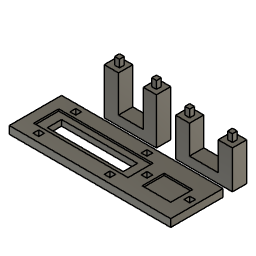
finalFrame_v1 (Autodesk Fusion 360 design; units mm, degrees)
Autodesk Fusion 360 part; units mm, degrees
sketch "草图1" plane through (0, 0, 0) normal (0, 0, 1) x (1, 0, 0)
  line L0 (0, 0) -> (-99.2, 0)
  line L1 (-99.2, 0) -> (-99.2, 26.2)
  line L2 (-99.2, 26.2) -> (0, 26.2)
  line L3 (0, 26.2) -> (0, 0)
  line L4 (15, 0) -> (45, 0)
  line L5 (45, 0) -> (45, 23)
  line L6 (45, 23) -> (15, 23)
  line L7 (15, 23) -> (15, 0)
  line L8 (5, 15) -> (10, 15)
  line L9 (10, 15) -> (10, 10)
  line L10 (10, 10) -> (5, 10)
  line L11 (5, 10) -> (5, 15)
  line L12 (50, 15) -> (55, 15)
  line L13 (55, 15) -> (55, 10)
  line L14 (55, 10) -> (50, 10)
  line L15 (50, 10) -> (50, 15)
  line L16 (-90, 35) -> (-85, 35)
  line L17 (-85, 35) -> (-85, 30)
  line L18 (-85, 30) -> (-90, 30)
  line L19 (-90, 30) -> (-90, 35)
  line L20 (-90, -4) -> (-85, -4)
  line L21 (-85, -4) -> (-85, -9)
  line L22 (-85, -9) -> (-90, -9)
  line L23 (-90, -9) -> (-90, -4)
  line L24 (-15, 35) -> (-10, 35)
  line L25 (-10, 35) -> (-10, 30)
  line L26 (-10, 30) -> (-15, 30)
  line L27 (-15, 30) -> (-15, 35)
  line L28 (-15, -9) -> (-10, -9)
  line L29 (-10, -9) -> (-10, -4)
  line L30 (-10, -4) -> (-15, -4)
  line L31 (-15, -4) -> (-15, -9)
  line L32 (-110, 40) -> (60, 40)
  line L33 (60, 40) -> (60, -15)
  line L34 (60, -15) -> (-110, -15)
  line L35 (-110, -15) -> (-110, 40)
  line L36 (-90, 20) -> (-10, 20)
  line L37 (-10, 20) -> (-10, 5)
  line L38 (-10, 5) -> (-90, 5)
  line L39 (-90, 5) -> (-90, 20)
  dimension "d1" = 26.2
  dimension "d2" = 99.2
  dimension "d3" = 23
  dimension "d4" = 30
  dimension "d5" = 5
  dimension "d6" = 5
  dimension "d7" = 55
  dimension "d8" = 170
  constraint horizontal L0
  constraint vertical L1
  constraint horizontal L2
  constraint vertical L3
  constraint coincident L0.start L3.end
  constraint horizontal L4
  constraint vertical L5
  constraint horizontal L6
  constraint vertical L7
  constraint horizontal L8
  constraint vertical L9
  constraint horizontal L10
  constraint vertical L11
  constraint horizontal L12
  constraint vertical L13
  constraint horizontal L14
  constraint vertical L15
  constraint horizontal L16
  constraint vertical L17
  constraint horizontal L18
  constraint vertical L19
  constraint horizontal L20
  constraint vertical L21
  constraint horizontal L22
  constraint vertical L23
  constraint horizontal L24
  constraint vertical L25
  constraint horizontal L26
  constraint vertical L27
  constraint horizontal L28
  constraint vertical L29
  constraint horizontal L30
  constraint vertical L31
  constraint horizontal L32
  constraint vertical L33
  constraint horizontal L34
  constraint vertical L35
  constraint horizontal L36
  constraint vertical L37
  constraint horizontal L38
  constraint vertical L39
  measures "d1" distance of L0.end L1.end
  measures "d2" distance of L1.end L2.end
  measures "d3" distance of L4.end L5.end
  measures "d4" distance of L5.end L6.end
  measures "d5" distance of L12.start L14.end
  measures "d6" distance of L12.start L12.end
  measures "d7" distance of L32.start L34.end
  measures "d8" distance of L32.start L32.end
sketch "草图2" plane through (0, 0, 0) normal (0, 0, 1) x (1, 0, 0)
  line L0 (-90, -9) -> (-85, -9)
  line L1 (-85, -9) -> (-85, -4)
  line L2 (-85, -4) -> (-90, -4)
  line L3 (-90, -4) -> (-90, -9)
  line L4 (-15, -9) -> (-10, -9)
  line L5 (-10, -9) -> (-10, -4)
  line L6 (-10, -4) -> (-15, -4)
  line L7 (-15, -4) -> (-15, -9)
  line L8 (-15, 30) -> (-10, 30)
  line L9 (-10, 30) -> (-10, 35)
  line L10 (-10, 35) -> (-15, 35)
  line L11 (-15, 35) -> (-15, 30)
  line L12 (-90, 30) -> (-85, 30)
  line L13 (-85, 30) -> (-85, 35)
  line L14 (-85, 35) -> (-90, 35)
  line L15 (-90, 35) -> (-90, 30)
  line L16 (-95, 26.2) -> (-80, 26.2)
  line L17 (-80, 26.2) -> (-80, 40)
  line L18 (-80, 40) -> (-95, 40)
  line L19 (-95, 40) -> (-95, 26.2)
  line L20 (-95, -15) -> (-80, -15)
  line L21 (-80, -15) -> (-80, 0)
  line L22 (-80, 0) -> (-95, 0)
  line L23 (-95, 0) -> (-95, -15)
  line L24 (-95, -15) -> (-80, -15)
  line L25 (-80, -15) -> (-80, 40)
  line L26 (-80, 40) -> (-95, 40)
  line L27 (-95, 40) -> (-95, -15)
  line L28 (-95, 0) -> (-80, 0)
  line L29 (-80, 0) -> (-80, 26.2)
  line L30 (-80, 26.2) -> (-95, 26.2)
  line L31 (-95, 26.2) -> (-95, 0)
  line L32 (5, 10) -> (10, 10)
  line L33 (10, 10) -> (10, 15)
  line L34 (10, 15) -> (5, 15)
  line L35 (5, 15) -> (5, 10)
  line L36 (50, 10) -> (55, 10)
  line L37 (55, 10) -> (55, 15)
  line L38 (55, 15) -> (50, 15)
  line L39 (50, 15) -> (50, 10)
  line L40 (0, 5) -> (15, 5)
  line L41 (15, 5) -> (15, 20)
  line L42 (15, 20) -> (0, 20)
  line L43 (0, 20) -> (0, 5)
  line L44 (45, 5) -> (60, 5)
  line L45 (60, 5) -> (60, 20)
  line L46 (60, 20) -> (45, 20)
  line L47 (45, 20) -> (45, 5)
  line L48 (0, 5) -> (60, 5)
  line L49 (60, 5) -> (60, 20)
  line L50 (60, 20) -> (0, 20)
  line L51 (0, 20) -> (0, 5)
  line L52 (15, 5) -> (45, 5)
  line L53 (45, 5) -> (45, 20)
  line L54 (45, 20) -> (15, 20)
  line L55 (15, 20) -> (15, 5)
  constraint horizontal L0
  constraint vertical L1
  constraint horizontal L2
  constraint vertical L3
  constraint horizontal L4
  constraint vertical L5
  constraint horizontal L6
  constraint vertical L7
  constraint horizontal L8
  constraint vertical L9
  constraint horizontal L10
  constraint vertical L11
  constraint horizontal L12
  constraint vertical L13
  constraint horizontal L14
  constraint vertical L15
  constraint horizontal L16
  constraint vertical L17
  constraint horizontal L18
  constraint vertical L19
  constraint horizontal L20
  constraint vertical L21
  constraint horizontal L22
  constraint vertical L23
  constraint horizontal L24
  constraint vertical L25
  constraint horizontal L26
  constraint vertical L27
  constraint horizontal L28
  constraint vertical L29
  constraint horizontal L30
  constraint vertical L31
  constraint horizontal L32
  constraint vertical L33
  constraint horizontal L34
  constraint vertical L35
  constraint horizontal L36
  constraint vertical L37
  constraint horizontal L38
  constraint vertical L39
  constraint horizontal L40
  constraint vertical L41
  constraint horizontal L42
  constraint vertical L43
  constraint horizontal L44
  constraint vertical L45
  constraint horizontal L46
  constraint vertical L47
  constraint horizontal L48
  constraint vertical L49
  constraint horizontal L50
  constraint vertical L51
  constraint horizontal L52
  constraint vertical L53
  constraint horizontal L54
  constraint vertical L55
extrude "拉伸1" add sketch "草图1" along normal blind 6 contours L0 L1 L2 L3 makes body 1
extrude "拉伸2" add sketch "草图1" along normal blind 8 contours L32 L33 L34 L35 bodies 1
extrude "拉伸3" add sketch "草图1" along normal blind 6 contours L4 L5 L6 L7 bodies 1
extrude "拉伸4" add sketch "草图2" against normal blind 10 separate body contours L16 L22 L25 L27 L28 L29 L30 L31 makes body 2
extrude "拉伸5" add sketch "草图2" against normal blind 48.5 contours L20 L21 L22 L23 L24 L25 L27 L28 bodies 2
extrude "拉伸6" add sketch "草图2" against normal blind 48.5 contours L16 L17 L18 L19 L25 L26 L27 L30 bodies 2
extrude "拉伸7" add sketch "草图2" against normal blind 56.5 contours L0 L1 L2 L3 bodies 2
extrude "拉伸8" add sketch "草图2" against normal blind 56.5 contours L12 L13 L14 L15 bodies 2
extrude "拉伸9" add sketch "草图2" against normal blind 10 separate body contours L41 L47 L48 L50 L52 L53 L54 L55 makes body 3
extrude "拉伸10" add sketch "草图2" against normal blind 48 separate body contours L32 L33 L34 L35 makes body 4
extrude "拉伸11" add sketch "草图2" against normal blind 48 separate body contours L36 L37 L38 L39 makes body 5
extrude "拉伸12" add sketch "草图2" against normal blind 40 contours L40 L41 L42 L43 L48 L50 L51 L55 bodies 3 4
extrude "拉伸13" add sketch "草图2" against normal blind 40 contours L44 L45 L46 L47 L48 L49 L50 L53 bodies 3 5
copy_body "复制和粘贴实体1" bodies 2 makes body 6
move_body "移动1" bodies 6 to x (1, 0, 0) y (0, 1, 0) z (0, 0, 1) at (0, 0, 0)
move_body "移动2" bodies 6 to x (1, 0, 0) y (0, 1, 0) z (0, 0, 1) at (70, 0, 0)
move_body "移动3" bodies 6 to x (1, 0, 0) y (0, 1, 0) z (0, 0, 1) at (5, 0, 0)
move_body "移动4" bodies 6 to x (-1, 0, 0) y (0, 1, 0) z (0, 0, -1) at (-40, 0, 0)
extrude "拉伸14" cut 1 faces at (-86.6667, 30, 2.6667) along direction (0, -1, 0) blind 0.5 on bodies 1 bodies 1
extrude "拉伸15" cut 1 faces at (-88.3333, 35, 2.6667) along direction (0, 1, 0) blind 0.5 on bodies 1 bodies 1
extrude "拉伸16" cut 1 faces at (-90, 31.5, 2.6667) along direction (-1, 0, 0) blind 0.5 on bodies 1 bodies 1
extrude "拉伸17" cut 1 faces at (-85, 33.5, 2.6667) along direction (1, 0, 0) blind 0.5 on bodies 1 bodies 1
extrude "拉伸18" cut 1 faces at (-13.3333, 35, 5.3333) along direction (0, 1, 0) blind 0.5 on bodies 1 bodies 1
extrude "拉伸19" cut 1 faces at (-15, 31.8333, 2.6667) along direction (-1, 0, 0) blind 0.5 on bodies 1 bodies 1
extrude "拉伸20" cut 1 faces at (-10, 33.6667, 2.6667) along direction (1, 0, 0) blind 0.5 on bodies 1 bodies 1
extrude "拉伸21" cut 1 faces at (-11.5, 30, 5.3333) along direction (0, -1, 0) blind 0.5 on bodies 1 bodies 1
extrude "拉伸22" cut 1 faces at (-90, -7.3333, 2.6667) along direction (-1, 0, 0) blind 0.5 on bodies 1 bodies 1
extrude "拉伸23" cut 1 faces at (-88.6667, -4, 2.6667) along direction (0, 1, 0) blind 0.5 on bodies 1 bodies 1
extrude "拉伸24" cut 1 faces at (-85, -5.3333, 5.3333) along direction (1, 0, 0) blind 0.5 on bodies 1 bodies 1
extrude "拉伸25" cut 1 faces at (-88.5, -9, 5.3333) along direction (0, -1, 0) blind 0.5 on bodies 1 bodies 1
extrude "拉伸26" cut 1 faces at (-10, -7.3333, 2.6667) along direction (1, 0, 0) blind 0.5 on bodies 1 bodies 1
extrude "拉伸27" cut 1 faces at (-13.1667, -9, 2.6667) along direction (0, -1, 0) blind 0.5 on bodies 1 bodies 1
extrude "拉伸28" cut 1 faces at (-15, -7.6667, 5.3333) along direction (-1, 0, 0) blind 0.5 on bodies 1 bodies 1
extrude "拉伸29" cut 1 faces at (-13.5, -4, 2.6667) along direction (0, 1, 0) blind 0.5 on bodies 1 bodies 1
extrude "拉伸30" cut 1 faces at (6.6667, 15, 5.3333) along direction (0, 1, 0) blind 0.5 on bodies 1 bodies 1
extrude "拉伸31" cut 1 faces at (5, 11.8333, 2.6667) along direction (-1, 0, 0) blind 0.5 on bodies 1 bodies 1
extrude "拉伸32" cut 1 faces at (51.6667, 15, 5.3333) along direction (0, 1, 0) blind 0.5 on bodies 1 bodies 1
extrude "拉伸33" cut 1 faces at (50, 11.8333, 2.6667) along direction (-1, 0, 0) blind 0.5 on bodies 1 bodies 1
extrude "拉伸34" cut 1 faces at (55, 13.6667, 2.6667) along direction (1, 0, 0) blind 0.5 on bodies 1 bodies 1
extrude "拉伸35" cut 1 faces at (53.5, 10, 5.3333) along direction (0, -1, 0) blind 0.5 on bodies 1 bodies 1
extrude "拉伸36" cut 1 faces at (10, 13.6667, 2.6667) along direction (1, 0, 0) blind 0.5 on bodies 1 bodies 1
extrude "拉伸37" cut 1 faces at (8.5, 10, 5.3333) along direction (0, -1, 0) blind 0.5 on bodies 1 bodies 1
extrude "拉伸38" cut 1 faces at (15, 10, -30) along direction (-1, 0, 0) blind 0.2 on bodies 3 bodies 3
extrude "拉伸39" cut 1 faces at (0, 15, -26.6667) along direction (1, 0, 0) blind 0.2 on bodies 3 bodies 3
copy_body "复制和粘贴实体2" bodies 3 makes body 7
move_body "移动5" bodies 7 to x (1, 0, 0) y (0, 1, 0) z (0, 0, 1) at (0, 0, 0)
move_body "移动6" bodies 7 to x (1, 0, 0) y (0, -1, 0) z (0, 0, -1) at (0, 40, 0)
move_body "移动7" bodies 7 to x (1, 0, 0) y (0, 1, 0) z (0, 0, 1) at (0, 30, 0)
move_body "移动8" bodies 6 to x (0, -1, 0) y (1, 0, 0) z (0, 0, 1) at (-60, 20, 0)
move_body "移动9" bodies 6 to x (1, 0, 0) y (0, 1, 0) z (0, 0, 1) at (0, 10, 0)
hidden bodies 2 3
